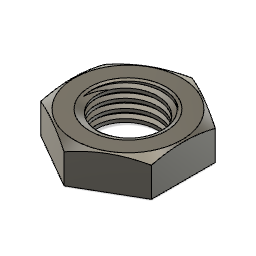
гайка 1 (Autodesk Fusion 360 design; units mm, degrees)
Autodesk Fusion 360 part; units mm, degrees
sketch "Sketch1" plane through (0, 0, 0) normal (0, 1, 0) x (1, 0, 0)
  line L0 (40, 23.094) -> (0, 46.188)
  line L1 (0, 46.188) -> (-40, 23.094)
  line L2 (-40, 23.094) -> (-40, -23.094)
  line L3 (-40, -23.094) -> (0, -46.188)
  line L4 (0, -46.188) -> (40, -23.094)
  line L5 (40, -23.094) -> (40, 23.094)
extrude "Extrude1" add sketch "Sketch1" along normal blind 25
hole "Hole1" at (0, 25, 0) direction (0, -1, 0) diameter 45.97 depth 30 tip angle 180
thread "Thread1" "ACME Screw Threads 2.0000 4G" major diameter 51.562 minor diameter 44.61 pitch 6.35 angle 29 modelled right hand crest width 2.3697 on face at (2.2886, 8.3333, 22.8708) crest through (0, 23.4125, 22.305)
ref_plane "WorkPlane1" through (40, 25, -23.094) normal (0.5, 0, 0.866025) x (0, 1, 0)
sketch "Sketch2" plane through (40, 25, -23.094) normal (0.5, 0, 0.866025) x (0, 1, 0)
  line L0 (1, 83) -> (-5, 95)
  line L1 (-5, 95) -> (3, 95)
  line L2 (3, 95) -> (1, 83)
  constraint horizontal L1
revolve "Revolve1" cut sketch "Sketch2" angle 360 about axis through (0, 1.75, 0) along (0, 1, 0)
sketch "Sketch4" plane through (40, 25, -23.094) normal (0.5, 0, 0.866025) x (0, 1, 0)
  line L0 (1, 76) -> (-3, 67)
  line L1 (-3, 67) -> (4.375, 67)
  line L2 (4.375, 67) -> (1, 76)
  constraint horizontal L1
revolve "Revolve2" cut sketch "Sketch4" angle 360 about axis through (0, 1.75, 0) along (0, 1, 0)
